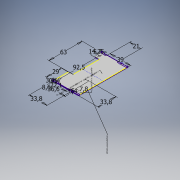
# Autodesk Inventor part: PlytkaWymiary
Saved by Autodesk Inventor 2019 (Build 230136000, 136)
## iProperties
Created: 2022-05-16
Part Number: PlytkaWymiary
Material: Ogólny
Document SubType Name: Modeling
Designer: Michał
Density: 1 g/cm^3
Appearance: Domyślna
Author: Michał
Autodesk Inventor part; units mm, degrees
ref_plane "YZ Plane" through (0, 0, 0) normal (1, 0, 0) x (0, 1, 0)
ref_plane "XZ Plane" through (0, 0, 0) normal (0, 1, 0) x (-1, 0, 0)
ref_plane "XY Plane" through (0, 0, 0) normal (0, 0, 1) x (1, 0, 0)
sketch "Szkic1" plane through (0, 0, 0) normal (0, 1, 0) x (-1, 0, 0)
  line L0 (0, 0) -> (39, 0)
  line L1 (39, 0) -> (39, -92.5)
  line L2 (39, -92.5) -> (0, -92.5)
  line L3 (0, -92.5) -> (0, 0)
  line L4 (39, 0) -> (47.6, 0)
  line L5 (47.6, 0) -> (47.6, -29)
  line L6 (47.6, -29) -> (39, -29)
  line L7 (39, -29) -> (39, 0)
  line L8 (0, -46.25) -> (39, -46.25) construction
  line L9 (0, 0) -> (7.8, 0) construction
  line L10 (7.8, 0) -> (7.8, -5) construction
  line L11 (7.8, -5) -> (0, -5) construction
  line L12 (0, -5) -> (0, 0) construction
  line L13 (0, -92.5) -> (7.8, -92.5) construction
  line L14 (7.8, -92.5) -> (7.8, -87.5) construction
  line L15 (7.8, -87.5) -> (0, -87.5) construction
  line L16 (0, -87.5) -> (0, -92.5) construction
  line L17 (39, -92.5) -> (47.6, -92.5)
  line L18 (47.6, -92.5) -> (47.6, -78.25)
  line L19 (47.6, -78.25) -> (39, -78.25)
  line L20 (39, -78.25) -> (39, -92.5)
  line L21 (39, -92.5) -> (18, -92.5) construction
  line L22 (18, -92.5) -> (18, -29.5) construction
  line L23 (18, -29.5) -> (39, -29.5) construction
  line L24 (39, -29.5) -> (39, -92.5) construction
  circle A0 centre (47.7, -0.5) radius 1.7
  circle A1 centre (11.1, -0.5) radius 1.7
  circle A2 centre (47.7, -92) radius 1.7
  circle A3 centre (11.1, -92) radius 1.7
  point P0 (13.8, -33.8)
  point P1 (13.8, -58.7)
  dimension "d0" = 39
  dimension "d1" = 92.5
  dimension "d2" = 8.6
  dimension "d3" = 29
  dimension "d4" = 33.8
  dimension "d5" = 33.8
  dimension "d6" = 5
  dimension "d7" = 7.8
  dimension "d9" = 14.25
  dimension "d10" = 63
  dimension "d11" = 21
  dimension "d12" = 0.1
  dimension "d13" = 3.4
  dimension "d14" = 0.5
  dimension "d15" = 36.6
  constraints: 50 end point, 10 parallel, 6 symmetric about line, 5 horizontal, 5 perpendicular, 4 centre point, 2 midpoint, 1 collinear, 1 equal radius, 1 horizontal alignment, 2 other
  measures "d0" distance of L1.end L2.end
  measures "d1" distance of L0.end L1.end
  measures "d2" distance of L0.end L4.end
  measures "d3" distance between parallel lines of L6 L4
  measures "d4" distance from line of L0 point (13.8, -33.8)
  measures "d5" distance from line of L5 point (13.8, -33.8)
  measures "d6" distance of L9.end L10.end
  measures "d7" distance of L10.end L11.end
  measures "d9" distance between parallel lines of L17 L19
  measures "d10" distance between parallel lines of L21 L23
  measures "d11" distance between parallel lines of L1 L22
  measures "d12" distance from line of L5 A0.centre
  measures "d13" diameter of A0
  measures "d14" distance from line of L4 A0.centre
  measures "d15" distance of A0.centre A1.centre
extrude "Plytka" add sketch "Szkic1" along normal blind 1 contours L0 A1 L1 L2 A3 L3 | L0 A1 | A3 L2 | L4 A0 L5 L6 L1 | L4 L5 A0 | L1 L19 L18 A2 L17 | A2 L18 L17 picked at (10.5661, -0.3857) picked at (10.6392, -91.3315) picked at (47.4739, -1.4428) picked at (47.4739, -91.0572)
extrude "Otwory" cut sketch "Szkic1" along normal up to surface (1 mm away) contours A1 L0 | L0 A1 | A3 L2 | L2 A3 | A0 L5 L4 | L4 L5 A0 | A2 L18 L17 | L17 L18 A2
sketch "Marginesy(Nie dotycza spodu plytki w strefie czujnika lini)" plane through (0, 1, 0) normal (0, 1, 0) x (1, 0, 0)
  line L0 (-47.6, 0) -> (-39, 0)
  line L1 (-39, 0) -> (-39, 2.4)
  line L2 (-39, 2.4) -> (-47.6, 2.4)
  line L3 (-47.6, 2.4) -> (-47.6, 0)
  line L4 (-46.0752, 0) -> (-12.7248, 0) projected
  line L5 (-47.6, 29) -> (-47.6, 2.1971) projected
  line L6 (-39, 78.25) -> (-39, 29) projected
  line L7 (-39, 0) -> (-16.9, 0)
  line L8 (-16.9, 0) -> (-16.9, 0.4)
  line L9 (-16.9, 0.4) -> (-39, 0.4)
  line L10 (-39, 0.4) -> (-39, 0)
  line L11 (0, 0) -> (0, 92.5) projected
  line L12 (-16.9, 0) -> (0, 0)
  line L13 (0, 0) -> (0, 2.4)
  line L14 (0, 2.4) -> (-16.9, 2.4)
  line L15 (-16.9, 2.4) -> (-16.9, 0)
  line L16 (0, 46.25) -> (-39, 46.25) construction
  line L17 (-47.6, 92.5) -> (-39, 92.5)
  line L18 (-39, 92.5) -> (-39, 90.1)
  line L19 (-39, 90.1) -> (-47.6, 90.1)
  line L20 (-47.6, 90.1) -> (-47.6, 92.5)
  line L21 (-46.0752, 92.5) -> (-12.7248, 92.5)
  line L22 (-39, 92.5) -> (-16.9, 92.5)
  line L23 (-16.9, 92.5) -> (-16.9, 92.1)
  line L24 (-16.9, 92.1) -> (-39, 92.1)
  line L25 (-39, 92.1) -> (-39, 92.5)
  line L26 (-16.9, 92.5) -> (0, 92.5)
  line L27 (0, 92.5) -> (0, 90.1)
  line L28 (0, 90.1) -> (-16.9, 90.1)
  line L29 (-16.9, 90.1) -> (-16.9, 92.5)
  arc A0 (-47.6, 90.3029) -> (-46.0752, 92.5) centre (-47.7, 92) ccw construction
  circle A1 centre (-47.7, 92) radius 2.85 construction
  arc A2 (-12.7248, 92.5) -> (-9.4752, 92.5) centre (-11.1, 92) ccw construction
  circle A3 centre (-11.1, 92) radius 2.85 construction
  arc A4 (-46.0752, 0) -> (-47.6, 2.1971) centre (-47.7, 0.5) ccw construction
  arc A5 (-9.4752, 0) -> (-12.7248, 0) centre (-11.1, 0.5) ccw construction
  circle A6 centre (-47.7, 0.5) radius 2.85 construction
  circle A7 centre (-11.1, 0.5) radius 2.85 construction
  point P0 (0, 92.5)
  dimension "d20" = 2.4
  dimension "d21" = 0.4
  dimension "d22" = 22.1
  dimension "d24" = 5.7
  constraints: 52 end point, 14 symmetric about line, 6 parallel, 4 centre point, 4 coincident, 4 collinear, 4 perpendicular, 3 equal radius, 3 horizontal, 2 point on line, 1 midpoint
  measures "d20" distance between parallel lines of L0 L2
  measures "d21" distance between parallel lines of L9 L4
  measures "d22" distance from line of L9.end L8
  measures "d24" diameter of A1
